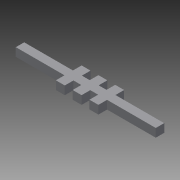
# Autodesk Inventor part: link1
Saved by Autodesk Inventor 2014 SP1 (Build 180222100, 222)
## iProperties
Created: 2015-02-17
Part Number: link1
Material: Generic
Document SubType Name: Modeling
Designer: Erin
Density: 1 g/cm^3
Appearance: Default
Author: Erin
Autodesk Inventor part; units mm, degrees
ref_plane "YZ Plane" through (0, 0, 0) normal (1, 0, 0) x (0, 1, 0)
ref_plane "XZ Plane" through (0, 0, 0) normal (0, 1, 0) x (-1, 0, 0)
ref_plane "XY Plane" through (0, 0, 0) normal (0, 0, 1) x (1, 0, 0)
sketch "tabs" plane through (0, 0, 0) normal (0, 0, 1) x (1, 0, 0)
  line L0 (16.0425, 13.6368) -> (18.7425, 13.6368)
  line L1 (18.7425, 13.6368) -> (18.7425, 10.7868)
  line L2 (18.7425, 10.7868) -> (16.0425, 10.7868)
  line L3 (16.0425, 10.7868) -> (16.0425, 13.6368)
  line L4 (22.0425, 13.6368) -> (24.7425, 13.6368)
  line L5 (24.7425, 13.6368) -> (24.7425, 10.7868)
  line L6 (24.7425, 10.7868) -> (22.0425, 10.7868)
  line L7 (22.0425, 10.7868) -> (22.0425, 13.6368)
  line L8 (28.0425, 13.6368) -> (30.7425, 13.6368)
  line L9 (30.7425, 13.6368) -> (30.7425, 10.7868)
  line L10 (30.7425, 10.7868) -> (28.0425, 10.7868)
  line L11 (28.0425, 10.7868) -> (28.0425, 13.6368)
  line L12 (23.3925, 10.7868) -> (23.3925, 8.8536) construction
  point P0 (23.3925, 12.1901)
  dimension "d2" = 2.7
  dimension "d3" = 3.3
  dimension "d4" = 3.3
  dimension "d5" = 2.85
  measures "d2" distance of L1.end L2.end
  measures "d3" distance between parallel lines of L7 L1
  measures "d4" distance between parallel lines of L11 L5
  measures "d5" distance of L2.end L0.start
sketch "Sketch1" plane through (0, 0, 0) normal (0, 0, 1) x (1, 0, 0)
  line L0 (-25, 1.5) -> (25, 1.5)
  line L1 (25, 1.5) -> (25, -1.5)
  line L2 (25, -1.5) -> (-25, -1.5)
  line L3 (-25, -1.5) -> (-25, 1.5)
  line L4 (0, 16.9043) -> (0, -20.0235) construction
  line L5 (-32.3473, 0) -> (40.4078, 0) construction
  line L6 (-7.35, 4.35) -> (-4.65, 4.35)
  line L7 (-4.65, 4.35) -> (-4.65, 1.5)
  line L8 (-4.65, 1.5) -> (-7.35, 1.5)
  line L9 (-7.35, 1.5) -> (-7.35, 4.35)
  line L10 (-1.35, 4.35) -> (1.35, 4.35)
  line L11 (1.35, 4.35) -> (1.35, 1.5)
  line L12 (1.35, 1.5) -> (-1.35, 1.5)
  line L13 (-1.35, 1.5) -> (-1.35, 4.35)
  line L14 (4.65, 4.35) -> (7.35, 4.35)
  line L15 (7.35, 4.35) -> (7.35, 1.5)
  line L16 (7.35, 1.5) -> (4.65, 1.5)
  line L17 (4.65, 1.5) -> (4.65, 4.35)
  line L18 (0, 1.5) -> (0, -0.4332) construction
  line L19 (-7.35, -1.5) -> (-4.65, -1.5)
  line L20 (-4.65, -1.5) -> (-4.65, -4.35)
  line L21 (-4.65, -4.35) -> (-7.35, -4.35)
  line L22 (-7.35, -4.35) -> (-7.35, -1.5)
  line L23 (-1.35, -1.5) -> (1.35, -1.5)
  line L24 (1.35, -1.5) -> (1.35, -4.35)
  line L25 (1.35, -4.35) -> (-1.35, -4.35)
  line L26 (-1.35, -4.35) -> (-1.35, -1.5)
  line L27 (4.65, -1.5) -> (7.35, -1.5)
  line L28 (7.35, -1.5) -> (7.35, -4.35)
  line L29 (7.35, -4.35) -> (4.65, -4.35)
  line L30 (4.65, -4.35) -> (4.65, -1.5)
  line L31 (0, -4.35) -> (0, -6.2832) construction
  point P0 (0, 0)
  point P1 (0, 1.5)
  point P2 (25, 0)
  dimension "d0" = 50
  dimension "d1" = 3
  constraints: 12 end point, 4 horizontal, 3 parallel, 3 vertical, 2 midpoint, 2 perpendicular, 1 horizontal alignment, 1 vertical alignment
  measures "d0" distance of L1.end L2.end
  measures "d1" distance of L0.end L1.end
extrude "Extrusion1" add sketch "Sketch1" along normal blind 3
equation "\"d2\" = mat + kerf"
equation "\"d3\" = mat - kerf"
equation "\"d4\" = mat - kerf"
equation "\"d5\" = mat + 0.5 * kerf"
equation "\"d1\" = mat"
equation "\"d6\" = mat"
equation "\"mat\" = 3"
equation "\"kerf\" = -0.3"
body "Solid1"
